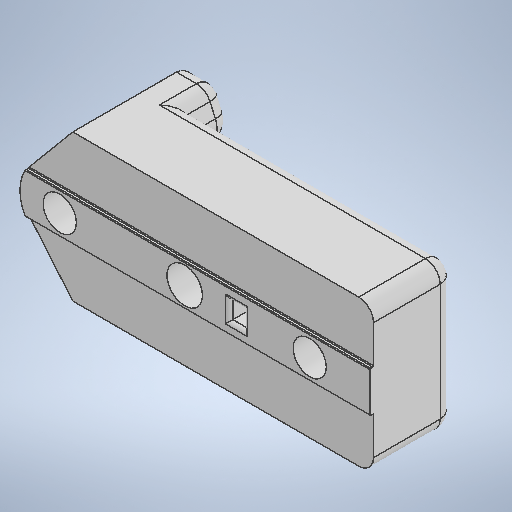
# Autodesk Inventor part: Base_Mount_Pivot
Saved by Autodesk Inventor 2026.2 (Build 302298000, 298)
## iProperties
Created: 2026-03-23
Part Number: Base_Mount_Pivot
Material: Generic
Document SubType Name: Modeling
Designer: Paco Ariel
Density: 1 g/cm^3
Appearance: Default
Author: Paco Ariel
Autodesk Inventor part; units mm, degrees
ref_plane "YZ Plane" through (0, 0, 0) normal (1, 0, 0) x (0, 1, 0)
ref_plane "XZ Plane" through (0, 0, 0) normal (0, 1, 0) x (-1, 0, 0)
ref_plane "XY Plane" through (0, 0, 0) normal (0, 0, 1) x (1, 0, 0)
sketch "Sketch1" plane through (0, 0, 0) normal (0, 0, 1) x (1, 0, 0)
  line L0 (-50, 19.775) -> (50, 19.775)
  line L1 (50, 19.775) -> (50, -19.775)
  line L2 (50, -19.775) -> (-50, -19.775)
  line L3 (-50, -19.775) -> (-50, 19.775)
  line L4 (-50, 19.775) -> (50, -19.775) construction
  line L5 (50, 19.775) -> (-50, -19.775) construction
  line L6 (50, -5.5) -> (-50, -5.5)
  line L7 (-50, -5.5) -> (-50, 5.5)
  line L8 (-50, 5.5) -> (50, 5.5)
  line L9 (50, 5.5) -> (50, -5.5)
  line L10 (50, -5.5) -> (-50, 5.5) construction
  line L11 (-50, -5.5) -> (50, 5.5) construction
  line L12 (33.75, 0) -> (-33.75, 0)
  circle A0 centre (-33.75, 0) radius 4.5
  circle A1 centre (33.75, 0) radius 4.5
  circle A2 centre (0, 0) radius 8
  point P0 (50, -5.5)
  point P1 (-5.8095, -5.5)
  point P2 (5.8095, -5.5)
  point P3 (5.8095, 5.5)
  point P4 (-5.8095, 5.5)
  dimension "d0" = 100
  dimension "d1" = 39.55
  dimension "d3" = 11
  dimension "d9" = 100
  dimension "d10" = 67.5
  dimension "d11" = 9
  dimension "d12" = 9
  dimension "d13" = 19.775
  dimension "d14" = 14.275
  dimension "d15" = 16
  constraints: 26 end point, 5 midpoint, 4 parallel, 3 centre point, 3 coincident, 3 horizontal, 2 perpendicular
  measures "d0" distance of L1.end L2.end
  measures "d1" distance of L0.end L1.end
  measures "d3" distance of L6.end L7.end
  measures "d9" distance between parallel lines of L9 L7
  measures "d10" distance of L12.start L12.end
  measures "d11" diameter of A0
  measures "d12" diameter of A1
  measures "d13" distance between parallel lines of L0 L12
  measures "d14" distance between parallel lines of L0 L8
  measures "d15" diameter of A2
extrude "Extrusion1" add sketch "Sketch1" along normal blind 1 contours L8 A2 L6 L3 | L1 L6 A2 L8 | L8 A2 L12 | A2 L12 L6
extrude "Extrusion2" add sketch "Sketch1" against normal blind 6
fillet "Fillet1" radius 0.2 4 edges at (0, 5.5, 0) (0, 5.5, 1) (0, -5.5, 1) (0, -5.5, 0)
sketch "Sketch2" plane through (0, 0, -6) normal (0, 0, -1) x (-1, 0, 0)
  circle A0 centre (33.75, 0) radius 4.5 projected
  circle A1 centre (-33.75, 0) radius 4.5 projected
  circle A2 centre (33.75, 0) radius 7
  circle A3 centre (-33.75, 0) radius 7
  line L0 (-50, -19.775) -> (50, -19.775) projected
  line L1 (-50, 19.775) -> (-50, -19.775) projected
  line L2 (50, 19.775) -> (-50, 19.775) projected
  line L3 (50, -19.775) -> (50, 19.775) projected
  point P0 (0, 0)
  dimension "d16" = 14
  dimension "d17" = 14
  constraints: 2 centre point, 2 coincident
  measures "d16" diameter of A2
  measures "d17" diameter of A3
extrude "Extrusion3" add sketch "Sketch2" along normal blind 16 contours L1 L2 L3 L0
sketch "Sketch3" plane through (0, 0, -22) normal (0, 0, -1) x (-1, 0, 0)
  circle A0 centre (0, 0) radius 5.15
  dimension "d21" = 10.3
  constraints: 1 centre point, 1 coincident
  measures "d21" diameter of A0
extrude "Extrusion4" cut sketch "Sketch3" against normal blind 10
sketch "Sketch4" plane through (0, 0, -22) normal (0, 0, -1) x (-1, 0, 0)
  circle A0 centre (0, 0) radius 5.15 projected
  circle A1 centre (0, 0) radius 7.25
  dimension "d24" = 14.5
  constraints: 1 centre point, 1 coincident
  measures "d24" diameter of A1
extrude "Extrusion5" add sketch "Sketch4" along normal blind 1
chamfer "Chamfer1" distance 1 distance2 1 1 edges at (7.25, 0, -22) measured on face at (7.75, 0, -22)
sketch "Sketch5" plane through (0, 0, -12) normal (0, 0, -1) x (-1, 0, 0)
  circle A0 centre (0, 0) radius 4.8
  dimension "d30" = 9.6
  constraints: 1 centre point, 1 coincident
  measures "d30" diameter of A0
extrude "Extrusion6" cut sketch "Sketch5" against normal blind 20
fillet "Fillet4" radius 4 4 edges at (50, -19.775, -11) (50, 19.775, -11) (-50, 19.775, -11) (-50, -19.775, -11)
sketch "Sketch7" plane through (0, 0, -22) normal (0, 0, -1) x (-1, 0, 0)
  circle A0 centre (-33.75, 0) radius 4.5 projected
  line L0 (-16, 2.5) -> (-16, -2.5)
  line L1 (0, 0) -> (-12, 0)
  line L2 (-12, 0) -> (-12, -2.5)
  line L3 (-12, -2.5) -> (-20, -2.5)
  line L4 (-20, -2.5) -> (-20, 2.5)
  line L5 (-20, 2.5) -> (-12, 2.5)
  line L6 (-12, 2.5) -> (-12, -2.5)
  dimension "d47" = 12
  dimension "d48" = 2.5
  dimension "d49" = 8
  dimension "d50" = 5
  dimension "d51" = 4
  constraints: 14 end point, 2 horizontal, 2 midpoint, 2 parallel, 2 vertical, 1 coincident, 1 perpendicular
  measures "d47" distance of L1.start L1.end
  measures "d48" distance of L1.end L2.end
  measures "d49" distance of L4.end L5.end
  measures "d50" distance of L3.end L4.end
  measures "d51" distance between parallel lines of L4 L0
extrude "Extrusion8" cut sketch "Sketch7" against normal blind 2 contours L0 L3 L4 L5
extrude "Extrusion9" cut sketch "Sketch7" against normal through all contours L5 L6 L2 L3 L0
sketch "Sketch8" plane through (0, 0, -22) normal (0, 0, -1) x (-1, 0, 0)
  circle A0 centre (0, 0) radius 4.8 projected
  circle A1 centre (0, 0) radius 23
  circle A2 centre (0, 0) radius 7.25 projected
  line L0 (0, 0) -> (38.5, 0)
  line L1 (38.5, 0) -> (13.5, 0)
  line L2 (13.5, 0) -> (13.5, -15.775)
  circle A3 centre (0, 0) radius 8.25 projected
  arc A4 (46, -19.775) -> (50, -15.775) centre (46, -15.775) ccw projected
  line L3 (50, -15.775) -> (50, 15.775) projected
  arc A5 (50, 15.775) -> (46, 19.775) centre (46, 15.775) ccw projected
  line L4 (46, 19.775) -> (-46, 19.775) projected
  arc A6 (-46, 19.775) -> (-50, 15.775) centre (-46, 15.775) ccw projected
  line L5 (-50, 15.775) -> (-50, -15.775) projected
  arc A7 (-50, -15.775) -> (-46, -19.775) centre (-46, -15.775) ccw projected
  line L6 (-46, -19.775) -> (46, -19.775) projected
  line L7 (-20, 2.5) -> (-12, 2.5) projected
  line L8 (-12, 2.5) -> (-12, -2.5) projected
  line L9 (-12, -2.5) -> (-20, -2.5) projected
  line L10 (-20, -2.5) -> (-20, 2.5) projected
  line L11 (17.75, 0) -> (33.75, 0)
  circle A8 centre (33.75, 0) radius 7 projected
  line L12 (42.9884, -23.359) -> (-29.2946, -23.359) construction
  line L13 (-29.2946, -23.359) -> (-29.2946, 22.5791) construction
  line L14 (-29.2946, 22.5791) -> (42.9884, 22.5791) construction
  line L15 (42.9884, 22.5791) -> (42.9884, -23.359) construction
  circle A9 centre (0, 0) radius 5.15 projected
  line L16 (19.7018, -11.8675) -> (23.2302, -19.775)
  arc A10 (41.9977, -6.8948) -> (41.9977, 6.8948) centre (33.75, 0) ccw
  line L17 (23.2302, -19.775) -> (31.2302, -19.775)
  line L18 (-46, -19.775) -> (46, -19.775) projected
  line L19 (31.2302, -19.775) -> (41.9977, -6.8948)
  line L20 (19.7018, 11.8675) -> (23.2302, 19.775)
  line L21 (23.2302, 19.775) -> (31.2302, 19.775)
  line L22 (31.2302, 19.775) -> (41.9977, 6.8948)
  point P0 (20.75, -9.9216)
  point P1 (23.0923, -19.775)
  dimension "d57" = 46
  dimension "d58" = 38.5
  dimension "d59" = 25
  dimension "d181" = 8
  constraints: 20 end point, 5 point on line, 4 point on circle, 4 symmetric about line, 2 centre point, 2 coincident, 1 collinear, 1 horizontal, 1 tangent, 1 vertical, 2 other
  measures "d57" diameter of A1
  measures "d58" distance of L0.start L0.end
  measures "d59" distance of L0.end L1.end
  measures "d181" distance of L16.end L17.end
fillet "Fillet6" radius 1 4 edges at (14, -2.5, 1) (12, 0, 1) (14, 2.5, 1) (16, 0, 1)
extrude "Extrusion10" cut sketch "Sketch8" against normal through all contours A0 | L4 A5 L3 A4 L6 L19 A10 L22
extrude "Extrusion11" add sketch "Sketch8" along normal blind 10 contours A1 L20 L4 L22 A10 L19 L6 L16
fillet "Fillet10" radius 5 2 edges at (-19.7018, -11.8675, -27) (-19.7018, 11.8675, -27)
fillet "Fillet11" radius 4 17 edges at (-23.2302, 19.775, -27) (-27.2302, 19.775, -32) (-20.2666, 12.0026, -32) (-23, 0, -32) (-20.2666, -12.0026, -32) (-21.9651, -16.9399, -32) (-21.9651, 16.9399, -32) (-44.5, 0, -32) (-36.6139, -13.3349, -32) (-36.6139, 13.3349, -32) (-27.2302, -19.775, -32) (-23.2302, -19.775, -27) (48.8284, -18.6034, -22) (50, 0, -22) (48.8284, 18.6034, -22) (11.3849, 19.775, -22) (11.3849, -19.775, -22)
equation "\"d9\" = d0"
body "Solid1"
